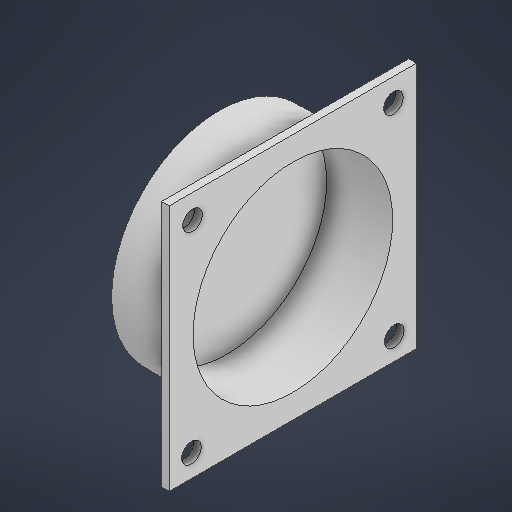
# Autodesk Inventor part: MagnetCap
Saved by Autodesk Inventor 2027 (Build 310192000, 192)
## iProperties
Created: 2026-06-10
Part Number: MagnetCap
Material: Generic
Document SubType Name: Modeling
Designer: giese
Density: 1 g/cm^3
Appearance: Default
Author: giese
Autodesk Inventor part; units mm, degrees
ref_plane "YZ Plane" through (0, 0, 0) normal (1, 0, 0) x (0, 1, 0)
ref_plane "XZ Plane" through (0, 0, 0) normal (0, 1, 0) x (-1, 0, 0)
ref_plane "XY Plane" through (0, 0, 0) normal (0, 0, 1) x (1, 0, 0)
sketch "Sketch1" plane through (0, 0, 0) normal (1, 0, 0) x (0, 1, 0)
  circle A0 centre (0, 0) radius 17.78
  dimension "d0" = 35.56
  constraints: 1 centre point, 1 coincident
  measures "d0" diameter of A0
extrude "Extrusion1" add sketch "Sketch1" along normal blind 1.27
sketch "Sketch2" plane through (1.27, 0, 0) normal (1, 0, 0) x (0, 0, -1)
  circle A0 centre (0, 0) radius 17.78
  circle A1 centre (0, 0) radius 16.51
  dimension "d3" = 35.56
  dimension "d4" = 33.02
  constraints: 2 centre point, 2 coincident
  measures "d3" diameter of A0
  measures "d4" diameter of A1
extrude "Extrusion2" add sketch "Sketch2" along normal blind 9.652
sketch "Sketch3" plane through (10.922, 0, 0) normal (1, 0, 0) x (0, 0, -1)
  line L0 (-20.45, -20.45) -> (20.45, -20.45)
  line L1 (20.45, -20.45) -> (20.45, 20.45)
  line L2 (20.45, 20.45) -> (-20.45, 20.45)
  line L3 (-20.45, 20.45) -> (-20.45, -20.45)
  line L4 (-20.45, -20.45) -> (20.45, 20.45) construction
  line L5 (20.45, -20.45) -> (-20.45, 20.45) construction
  point P0 (0, 0)
  dimension "d7" = 40.9
  dimension "d8" = 40.9
  constraints: 12 end point, 2 midpoint, 2 parallel, 1 horizontal, 1 perpendicular
  measures "d7" distance between parallel lines of L0 L2
  measures "d8" distance between parallel lines of L1 L3
extrude "Extrusion3" add sketch "Sketch3" along normal blind 1.27
sketch "Sketch4" plane through (12.192, 0, 0) normal (1, 0, 0) x (0, 0, -1)
  circle A0 centre (0, 0) radius 16.51
  line L0 (-20.45, 20.45) -> (-20.45, -20.45) projected
  line L1 (20.45, -20.45) -> (20.45, 20.45) projected
  line L2 (-20.45, -20.45) -> (20.45, -20.45) projected
  line L3 (20.45, 20.45) -> (-20.45, 20.45) projected
  line L4 (-16.7742, -16.7449) -> (16.7742, -16.745)
  line L5 (16.7742, -16.745) -> (16.7742, 16.745)
  line L6 (16.7742, 16.745) -> (-16.7742, 16.7449)
  line L7 (-16.7742, 16.7449) -> (-16.7742, -16.7449)
  line L8 (-16.7742, -16.7449) -> (16.7742, 16.745) construction
  line L9 (16.7742, -16.745) -> (-16.7742, 16.7449) construction
  circle A1 centre (-16.7742, -16.7449) radius 1.6262
  circle A2 centre (16.7687, -16.8222) radius 1.6262
  circle A3 centre (16.6447, 16.6573) radius 1.6262
  circle A4 centre (-16.5868, 16.4713) radius 1.6262
  dimension "d18" = 33.02
  dimension "d25" = 40.9
  dimension "d32" = 33.4899
  dimension "d33" = 33.5483
  dimension "d34" = 3.2524
  dimension "d35" = 3.2524
  dimension "d36" = 3.2524
  dimension "d37" = 3.2524
  constraints: 12 end point, 5 centre point, 2 coincident, 2 midpoint, 2 parallel, 1 horizontal, 1 perpendicular
  measures "d18" diameter of A0
  measures "d25" distance between parallel lines of L1 L0
  measures "d32" distance of L6.end L4.start
  measures "d33" distance of L5.end L6.end
  measures "d34" diameter of A1
  measures "d35" diameter of A2
  measures "d36" diameter of A3
  measures "d37" diameter of A4
extrude "Extrusion4" cut sketch "Sketch4" against normal blind 3.2524 contours A0 | L7 A1 L4 | L4 A1 L7 | A2 L5 L4 | L4 L5 A2 | A4 L6 L7 | L7 L6 A4 | A3 L6 L5 | L5 L6 A3
fillet "Fillet1" radius 1.778 1 edges at (10.922, 0, 17.78)
sketch "Sketch5" plane through (0, 0, 0) normal (-1, 0, 0) x (0, 0, 1)
  point P0 (0, 0)
equation "\"d16\" = d35"
body "Solid1"
